Autodesk Fusion 360 part; units mm, degrees
(part 6 of 14)
  arc A1361 (82.693, 15.5542) -> (82.693, 15.6558) centre (82.693, 15.605) ccw
  line L2871 (81.2795, 39.751) -> (80.8045, 39.751)
  arc A1362 (84.693, 13.5542) -> (84.693, 13.6558) centre (84.693, 13.605) ccw
  arc A1363 (82.7386, 13.3061) -> (82.7386, 13.0751) centre (82.7386, 13.1906) ccw
  line L2872 (84.193, 13.3675) -> (84.193, 13.8425)
  line L2873 (81.542, 40.5135) -> (81.542, 40.9885)
  line L2874 (82.042, 39.201) -> (82.042, 40.301)
  line L2875 (83.2795, 40.251) -> (82.8045, 40.251)
  line L2876 (83.2795, 39.251) -> (82.8045, 39.251)
  line L2877 (83.042, 38.751) -> (83.042, 40.751)
  arc A1364 (83.042, 38.7002) -> (83.042, 38.8018) centre (83.042, 38.751) ccw
  line L2878 (81.542, 38.5135) -> (81.542, 38.9885)
  arc A1365 (81.042, 40.7002) -> (81.042, 40.8018) centre (81.042, 40.751) ccw
  line L2879 (82.542, 40.5135) -> (82.542, 40.9885)
  line L2880 (82.542, 38.5135) -> (82.542, 38.9885)
  line L2881 (83.2795, 40.251) -> (82.8045, 40.251)
  arc A1366 (84.693, 13.6558) -> (84.693, 13.5542) centre (84.693, 13.605) ccw
  line L2882 (75.3115, 40.124) -> (75.7865, 40.124)
  line L2883 (82.042, 40.5135) -> (82.042, 40.9885)
  line L2884 (83.2795, 39.251) -> (82.8045, 39.251)
  line L2885 (82.042, 38.5135) -> (82.042, 38.9885)
  line L2886 (83.2795, 39.751) -> (82.8045, 39.751)
  line L2887 (83.2795, 40.251) -> (82.8045, 40.251)
  line L2888 (82.042, 40.5135) -> (82.042, 40.9885)
  line L2889 (82.042, 38.5135) -> (82.042, 38.9885)
  line L2890 (81.542, 40.5135) -> (81.542, 40.9885)
  line L2891 (82.042, 39.201) -> (82.042, 40.301)
  arc A1367 (81.042, 38.7002) -> (81.042, 38.8018) centre (81.042, 38.751) ccw
  line L2892 (83.193, 13.3675) -> (83.193, 13.8425)
  line L2893 (82.542, 38.5135) -> (82.542, 38.9885)
  arc A1368 (83.042, 38.8018) -> (83.042, 38.7002) centre (83.042, 38.751) ccw
  line L2894 (81.2795, 40.251) -> (80.8045, 40.251)
  line L2895 (84.693, 15.605) -> (82.693, 15.605)
  line L2896 (81.2795, 39.751) -> (80.8045, 39.751)
  line L2897 (82.042, 39.201) -> (82.042, 40.301)
  arc A1369 (81.0876, 38.4521) -> (81.0876, 38.2211) centre (81.0876, 38.3366) ccw
  line L2898 (81.542, 40.5135) -> (81.542, 40.9885)
  line L2899 (74.549, 38.8615) -> (74.549, 38.3865)
  line L2900 (81.042, 38.751) -> (83.042, 38.751)
  line L2901 (82.542, 38.5135) -> (82.542, 38.9885)
  line L2902 (81.2795, 39.251) -> (80.8045, 39.251)
  line L2903 (83.693, 13.3675) -> (83.693, 13.8425)
  line L2904 (83.2795, 39.751) -> (82.8045, 39.751)
  line L2905 (73.4385, 13.724) -> (73.9135, 13.724)
  line L2906 (84.9305, 15.105) -> (84.4555, 15.105)
  line L2907 (73.676, 15.224) -> (73.676, 13.224)
  line L2908 (74.676, 15.4615) -> (74.676, 14.9865)
  line L2909 (84.9305, 14.605) -> (84.4555, 14.605)
  arc A1370 (75.676, 15.1732) -> (75.676, 15.2748) centre (75.676, 15.224) ccw
  arc A1371 (73.676, 13.1732) -> (73.676, 13.2748) centre (73.676, 13.224) ccw
  line L2910 (81.2795, 39.751) -> (80.8045, 39.751)
  line L2911 (74.176, 13.4615) -> (74.176, 12.9865)
  line L2912 (82.9305, 14.105) -> (82.4555, 14.105)
  line L2913 (75.676, 13.224) -> (75.676, 15.224)
  line L2914 (83.693, 15.3675) -> (83.693, 15.8425)
  line L2915 (83.693, 13.3675) -> (83.693, 13.8425)
  line L2916 (84.9305, 14.105) -> (84.4555, 14.105)
  line L2917 (83.193, 15.3675) -> (83.193, 15.8425)
  line L2918 (73.4385, 14.724) -> (73.9135, 14.724)
  line L2919 (84.193, 13.3675) -> (84.193, 13.8425)
  line L2920 (84.9305, 14.605) -> (84.4555, 14.605)
  line L2921 (74.176, 15.4615) -> (74.176, 14.9865)
  line L2922 (81.2795, 40.251) -> (80.8045, 40.251)
  arc A1372 (73.676, 13.2748) -> (73.676, 13.1732) centre (73.676, 13.224) ccw
  line L2923 (73.4385, 14.724) -> (73.9135, 14.724)
  arc A1373 (75.676, 15.2748) -> (75.676, 15.1732) centre (75.676, 15.224) ccw
  line L2924 (82.9305, 14.605) -> (82.4555, 14.605)
  line L2925 (74.176, 15.4615) -> (74.176, 14.9865)
  line L2926 (74.176, 15.4615) -> (74.176, 14.9865)
  line L2927 (75.176, 15.4615) -> (75.176, 14.9865)
  arc A1374 (75.676, 13.2748) -> (75.676, 13.1732) centre (75.676, 13.224) ccw
  arc A1375 (73.676, 15.2748) -> (73.676, 15.1732) centre (73.676, 15.224) ccw
  line L2928 (75.176, 15.4615) -> (75.176, 14.9865)
  line L2929 (83.693, 14.055) -> (83.693, 15.155)
  line L2930 (82.693, 13.605) -> (84.693, 13.605)
  line L2931 (82.693, 15.605) -> (82.693, 13.605)
  arc A1376 (73.676, 15.1732) -> (73.676, 15.2748) centre (73.676, 15.224) ccw
  line L2932 (74.676, 15.4615) -> (74.676, 14.9865)
  line L2933 (83.193, 15.3675) -> (83.193, 15.8425)
  line L2934 (83.693, 15.3675) -> (83.693, 15.8425)
  arc A1377 (84.693, 15.6558) -> (84.693, 15.5542) centre (84.693, 15.605) ccw
  line L2935 (84.693, 13.605) -> (84.693, 15.605)
  line L2936 (84.9305, 14.105) -> (84.4555, 14.105)
  line L2937 (84.9305, 14.105) -> (84.4555, 14.105)
  line L2938 (82.9305, 14.105) -> (82.4555, 14.105)
  line L2939 (84.193, 15.3675) -> (84.193, 15.8425)
  line L2940 (83.693, 14.055) -> (83.693, 15.155)
  line L2941 (82.9305, 15.105) -> (82.4555, 15.105)
  line L2942 (84.193, 15.3675) -> (84.193, 15.8425)
  line L2943 (84.9305, 15.105) -> (84.4555, 15.105)
  line L2944 (83.693, 15.3675) -> (83.693, 15.8425)
  line L2945 (84.193, 13.3675) -> (84.193, 13.8425)
  arc A1378 (82.693, 13.5542) -> (82.693, 13.6558) centre (82.693, 13.605) ccw
  line L2946 (84.193, 15.3675) -> (84.193, 15.8425)
  line L2947 (82.9305, 14.105) -> (82.4555, 14.105)
  line L2948 (81.2795, 39.251) -> (80.8045, 39.251)
  line L2949 (84.9305, 14.605) -> (84.4555, 14.605)
  arc A1379 (84.693, 15.5542) -> (84.693, 15.6558) centre (84.693, 15.605) ccw
  line L2950 (82.9305, 15.105) -> (82.4555, 15.105)
  line L2951 (82.9305, 14.605) -> (82.4555, 14.605)
  line L2952 (82.9305, 14.605) -> (82.4555, 14.605)
  line L2953 (84.9305, 15.105) -> (84.4555, 15.105)
  line L2954 (83.693, 14.055) -> (83.693, 15.155)
  line L2955 (83.193, 15.3675) -> (83.193, 15.8425)
  line L2956 (73.4385, 14.224) -> (73.9135, 14.224)
  arc A1380 (82.693, 15.6558) -> (82.693, 15.5542) centre (82.693, 15.605) ccw
  line L2957 (82.9305, 15.105) -> (82.4555, 15.105)
  line L2958 (75.4385, 13.724) -> (75.9135, 13.724)
  line L2959 (92.629, 51.9281) -> (92.629, 52.9281)
  line L2960 (75.4385, 13.724) -> (75.9135, 13.724)
  line L2961 (91.723, 40.621) -> (91.723, 41.001)
  line L2962 (92.173, 39.771) -> (92.173, 40.151)
  line L2963 (92.104, 51.8131) -> (92.104, 52.1931)
  line L2964 (74.676, 15.4615) -> (74.676, 14.9865)
  line L2965 (75.176, 13.4615) -> (75.176, 12.9865)
  arc A1381 (75.6304, 15.7539) -> (75.6304, 15.5229) centre (75.6304, 15.6384) ccw
  line L2966 (92.554, 52.6631) -> (92.554, 53.0431)
  line L2967 (92.029, 52.7281) -> (92.629, 52.7281)
  line L2968 (74.676, 14.774) -> (74.676, 13.674)
  line L2969 (75.4385, 14.224) -> (75.9135, 14.224)
  line L2970 (92.248, 40.886) -> (91.648, 40.886)
  line L2971 (75.676, 15.224) -> (73.676, 15.224)
  line L2972 (74.176, 13.4615) -> (74.176, 12.9865)
  line L2973 (73.4385, 13.724) -> (73.9135, 13.724)
  line L2974 (92.104, 51.8131) -> (92.104, 52.1931)
  line L2975 (91.902, 22.979) -> (91.902, 21.979)
  line L2976 (92.173, 40.621) -> (92.173, 41.001)
  line L2977 (74.676, 13.4615) -> (74.676, 12.9865)
  arc A1382 (92.448, 39.986) -> (92.648, 39.986) centre (92.548, 39.986) ccw
  line L2978 (92.104, 52.6631) -> (92.104, 53.0431)
  line L2979 (91.902, 22.779) -> (92.502, 22.779)
  line L2980 (91.902, 21.979) -> (92.502, 21.979)
  line L2981 (92.104, 51.8131) -> (92.104, 52.1931)
  line L2982 (91.648, 40.686) -> (92.248, 40.686)
  line L2983 (91.723, 40.621) -> (91.723, 41.001)
  line L2984 (73.4385, 14.224) -> (73.9135, 14.224)
  line L2985 (73.4385, 13.724) -> (73.9135, 13.724)
  line L2986 (91.648, 39.886) -> (92.248, 39.886)
  line L2987 (74.676, 13.4615) -> (74.676, 12.9865)
  line L2988 (75.4385, 13.724) -> (75.9135, 13.724)
  line L2989 (75.4385, 14.224) -> (75.9135, 14.224)
  line L2990 (75.4385, 14.724) -> (75.9135, 14.724)
  line L2991 (74.176, 13.4615) -> (74.176, 12.9865)
  line L2992 (74.676, 14.774) -> (74.676, 13.674)
  arc A1383 (75.6304, 15.5229) -> (75.6304, 15.7539) centre (75.6304, 15.6384) ccw
  line L2993 (73.4385, 14.224) -> (73.9135, 14.224)
  line L2994 (73.4385, 14.724) -> (73.9135, 14.724)
  line L2995 (91.648, 40.886) -> (91.648, 39.886)
  arc A1384 (92.648, 39.986) -> (92.448, 39.986) centre (92.548, 39.986) ccw
  line L2996 (92.173, 39.771) -> (92.173, 40.151)
  line L2997 (74.676, 14.774) -> (74.676, 13.674)
  line L2998 (75.176, 13.4615) -> (75.176, 12.9865)
  line L2999 (92.029, 51.9281) -> (92.629, 51.9281)
  line L3000 (92.554, 52.6631) -> (92.554, 53.0431)
  line L3001 (91.723, 39.771) -> (91.723, 40.151)
  arc A1385 (93.029, 52.0281) -> (92.829, 52.0281) centre (92.929, 52.0281) ccw
  line L3002 (92.248, 39.886) -> (92.248, 40.886)
  line L3003 (75.4385, 14.724) -> (75.9135, 14.724)
  arc A1386 (75.676, 13.1732) -> (75.676, 13.2748) centre (75.676, 13.224) ccw
  line L3004 (92.173, 40.621) -> (92.173, 41.001)
  line L3005 (92.554, 52.6631) -> (92.554, 53.0431)
  line L3006 (92.173, 39.771) -> (92.173, 40.151)
  line L3007 (75.4385, 14.724) -> (75.9135, 14.724)
  line L3008 (92.554, 51.8131) -> (92.554, 52.1931)
  line L3009 (75.4385, 14.224) -> (75.9135, 14.224)
  line L3010 (91.648, 40.786) -> (92.248, 40.786)
  line L3011 (75.176, 13.4615) -> (75.176, 12.9865)
  line L3012 (73.676, 13.224) -> (75.676, 13.224)
  line L3013 (74.676, 13.4615) -> (74.676, 12.9865)
  line L3014 (75.176, 15.4615) -> (75.176, 14.9865)
  line L3015 (92.104, 52.6631) -> (92.104, 53.0431)
  arc A1387 (43.735, 39.8716) -> (43.735, 40.1383) centre (43.735, 40.005) ccw
  line L3016 (62.005, 17.735) -> (38.465, 17.735)
  arc A1388 (40.735, 39.8716) -> (40.735, 40.1383) centre (40.735, 40.005) ccw
  arc A1389 (37.8892, 40.2746) -> (37.2672, 40.2746) centre (37.5782, 40.2746) ccw
  arc A1390 (39.2088, 40.0206) -> (40.2656, 40.0206) centre (39.7372, 40.0206) ccw
  arc A1391 (92.829, 52.0281) -> (93.029, 52.0281) centre (92.929, 52.0281) ccw
  arc A1392 (42.735, 39.8716) -> (42.735, 40.1383) centre (42.735, 40.005) ccw
  arc A1393 (39.735, 40.1383) -> (39.735, 39.8717) centre (39.735, 40.005) ccw
  line L3017 (64.205, 15.535) -> (64.205, 43.475)
  arc A1394 (41.735, 40.1383) -> (41.735, 39.8717) centre (41.735, 40.005) ccw
  line L3018 (91.723, 39.771) -> (91.723, 40.151)
  line L3019 (92.104, 52.6631) -> (92.104, 53.0431)
  line L3020 (92.502, 22.979) -> (91.902, 22.979)
  line L3021 (92.681, 7.767) -> (92.681, 8.147)
  line L3022 (92.156, 8.682) -> (92.756, 8.682)
  line L3023 (91.723, 39.771) -> (91.723, 40.151)
  line L3024 (92.156, 8.882) -> (92.156, 7.882)
  line L3025 (92.756, 8.882) -> (92.156, 8.882)
  line L3026 (92.427, 21.864) -> (92.427, 22.244)
  line L3027 (92.681, 8.617) -> (92.681, 8.997)
  line L3028 (92.681, 7.767) -> (92.681, 8.147)
  line L3029 (92.427, 22.714) -> (92.427, 23.094)
  line L3030 (92.156, 8.782) -> (92.756, 8.782)
  line L3031 (92.756, 7.882) -> (92.756, 8.882)
  line L3032 (92.681, 8.617) -> (92.681, 8.997)
  arc A1395 (40.735, 39.8716) -> (40.735, 40.1383) centre (40.735, 40.005) ccw
  line L3033 (92.173, 40.621) -> (92.173, 41.001)
  line L3034 (92.681, 8.617) -> (92.681, 8.997)
  line L3035 (92.502, 21.979) -> (92.502, 22.979)
  arc A1396 (42.735, 39.8716) -> (42.735, 40.1383) centre (42.735, 40.005) ccw
  arc A1397 (92.956, 7.982) -> (93.156, 7.982) centre (93.056, 7.982) ccw
  line L3036 (92.029, 52.9281) -> (92.029, 51.9281)
  line L3037 (91.977, 21.864) -> (91.977, 22.244)
  line L3038 (92.231, 8.617) -> (92.231, 8.997)
  arc A1398 (41.735, 40.1383) -> (41.735, 39.8717) centre (41.735, 40.005) ccw
  line L3039 (92.156, 7.882) -> (92.756, 7.882)
  line L3040 (91.977, 21.864) -> (91.977, 22.244)
  line L3041 (64.205, 43.475) -> (36.265, 43.475)
  line L3042 (91.977, 22.714) -> (91.977, 23.094)
  line L3043 (92.231, 7.767) -> (92.231, 8.147)
  line L3044 (36.265, 15.535) -> (64.205, 15.535)
  arc A1399 (92.702, 22.079) -> (92.902, 22.079) centre (92.802, 22.079) ccw
  arc A1400 (41.735, 39.8716) -> (41.735, 40.1383) centre (41.735, 40.005) ccw
  line L3045 (91.723, 40.621) -> (91.723, 41.001)
  line L3046 (92.427, 21.864) -> (92.427, 22.244)
  line L3047 (91.902, 22.879) -> (92.502, 22.879)
  line L3048 (92.427, 22.714) -> (92.427, 23.094)
  line L3049 (92.681, 7.767) -> (92.681, 8.147)
  line L3050 (92.231, 8.617) -> (92.231, 8.997)
  arc A1401 (40.735, 40.1383) -> (40.735, 39.8717) centre (40.735, 40.005) ccw
  line L3051 (92.554, 51.8131) -> (92.554, 52.1931)
  line L3052 (92.231, 7.767) -> (92.231, 8.147)
  line L3053 (92.554, 51.8131) -> (92.554, 52.1931)
  arc A1402 (92.902, 22.079) -> (92.702, 22.079) centre (92.802, 22.079) ccw
  line L3054 (91.977, 22.714) -> (91.977, 23.094)
  line L3055 (92.427, 21.864) -> (92.427, 22.244)
  line L3056 (92.029, 52.8281) -> (92.629, 52.8281)
  line L3057 (91.977, 22.714) -> (91.977, 23.094)
  line L3058 (92.231, 8.617) -> (92.231, 8.997)
  arc A1403 (93.156, 7.982) -> (92.956, 7.982) centre (93.056, 7.982) ccw
  line L3059 (92.427, 22.714) -> (92.427, 23.094)
  line L3060 (48.395, 52.0775) -> (48.395, 54.3505)
  line L3061 (91.977, 21.864) -> (91.977, 22.244)
  line L3062 (92.629, 52.9281) -> (92.029, 52.9281)
  arc A1404 (44.735, 40.1383) -> (44.735, 39.8717) centre (44.735, 40.005) ccw
  arc A1405 (46.735, 39.8716) -> (46.735, 40.1383) centre (46.735, 40.005) ccw
  arc A1406 (48.735, 39.8716) -> (48.735, 40.1383) centre (48.735, 40.005) ccw
  arc A1407 (43.735, 39.8716) -> (43.735, 40.1383) centre (43.735, 40.005) ccw
  arc A1408 (47.735, 40.1383) -> (47.735, 39.8717) centre (47.735, 40.005) ccw
  arc A1409 (48.735, 40.1383) -> (48.735, 39.8717) centre (48.735, 40.005) ccw
  arc A1410 (43.735, 39.8716) -> (43.735, 40.1383) centre (43.735, 40.005) ccw
  arc A1411 (45.735, 39.8716) -> (45.735, 40.1383) centre (45.735, 40.005) ccw
  arc A1412 (45.735, 39.8716) -> (45.735, 40.1383) centre (45.735, 40.005) ccw
  arc A1413 (41.735, 39.8716) -> (41.735, 40.1383) centre (41.735, 40.005) ccw
  arc A1414 (47.735, 40.1383) -> (47.735, 39.8717) centre (47.735, 40.005) ccw
  arc A1415 (47.735, 39.8716) -> (47.735, 40.1383) centre (47.735, 40.005) ccw
  arc A1416 (42.735, 40.1383) -> (42.735, 39.8717) centre (42.735, 40.005) ccw
  arc A1417 (45.735, 40.1383) -> (45.735, 39.8717) centre (45.735, 40.005) ccw
  arc A1418 (43.735, 40.1383) -> (43.735, 39.8717) centre (43.735, 40.005) ccw
  arc A1419 (45.735, 40.1383) -> (45.735, 39.8717) centre (45.735, 40.005) ccw
  arc A1420 (37.2672, 40.2746) -> (37.8892, 40.2746) centre (37.5782, 40.2746) ccw
  arc A1421 (48.735, 39.8716) -> (48.735, 40.1383) centre (48.735, 40.005) ccw
  arc A1422 (49.735, 39.8716) -> (49.735, 40.1383) centre (49.735, 40.005) ccw
  arc A1423 (39.735, 39.8716) -> (39.735, 40.1383) centre (39.735, 40.005) ccw
  line L3063 (38.465, 17.735) -> (38.465, 41.275)
  arc A1424 (44.735, 40.1383) -> (44.735, 39.8717) centre (44.735, 40.005) ccw
  arc A1425 (39.735, 40.1383) -> (39.735, 39.8717) centre (39.735, 40.005) ccw
  arc A1426 (44.735, 39.8716) -> (44.735, 40.1383) centre (44.735, 40.005) ccw
  arc A1427 (49.735, 40.1383) -> (49.735, 39.8717) centre (49.735, 40.005) ccw
  arc A1428 (45.735, 40.1383) -> (45.735, 39.8717) centre (45.735, 40.005) ccw
  arc A1429 (46.735, 40.1383) -> (46.735, 39.8717) centre (46.735, 40.005) ccw
  arc A1430 (49.735, 39.8716) -> (49.735, 40.1383) centre (49.735, 40.005) ccw
  arc A1431 (42.735, 40.1383) -> (42.735, 39.8717) centre (42.735, 40.005) ccw
  arc A1432 (49.735, 40.1383) -> (49.735, 39.8717) centre (49.735, 40.005) ccw
  arc A1433 (49.735, 39.8716) -> (49.735, 40.1383) centre (49.735, 40.005) ccw
  arc A1434 (48.735, 40.1383) -> (48.735, 39.8717) centre (48.735, 40.005) ccw
  arc A1435 (46.735, 39.8716) -> (46.735, 40.1383) centre (46.735, 40.005) ccw
  arc A1436 (46.735, 40.1383) -> (46.735, 39.8717) centre (46.735, 40.005) ccw
  arc A1437 (40.735, 40.1383) -> (40.735, 39.8717) centre (40.735, 40.005) ccw
  arc A1438 (50.735, 39.8716) -> (50.735, 40.1383) centre (50.735, 40.005) ccw
  arc A1439 (44.735, 39.8716) -> (44.735, 40.1383) centre (44.735, 40.005) ccw
  arc A1440 (47.735, 39.8716) -> (47.735, 40.1383) centre (47.735, 40.005) ccw
  arc A1441 (48.735, 39.8716) -> (48.735, 40.1383) centre (48.735, 40.005) ccw
  arc A1442 (40.735, 39.8716) -> (40.735, 40.1383) centre (40.735, 40.005) ccw
  line L3064 (92.231, 7.767) -> (92.231, 8.147)
  arc A1443 (41.735, 40.1383) -> (41.735, 39.8717) centre (41.735, 40.005) ccw
  line L3065 (62.005, 41.275) -> (62.005, 17.735)
  arc A1444 (42.735, 39.8716) -> (42.735, 40.1383) centre (42.735, 40.005) ccw
  arc A1445 (43.735, 40.1383) -> (43.735, 39.8717) centre (43.735, 40.005) ccw
  arc A1446 (45.735, 39.8716) -> (45.735, 40.1383) centre (45.735, 40.005) ccw
  line L3066 (36.265, 43.475) -> (36.265, 15.535)
  arc A1447 (46.735, 40.1383) -> (46.735, 39.8717) centre (46.735, 40.005) ccw
  arc A1448 (40.2656, 40.0206) -> (39.2088, 40.0206) centre (39.7372, 40.0206) ccw
  arc A1449 (47.735, 39.8716) -> (47.735, 40.1383) centre (47.735, 40.005) ccw
  arc A1450 (41.735, 39.8716) -> (41.735, 40.1383) centre (41.735, 40.005) ccw
  arc A1451 (39.735, 39.8716) -> (39.735, 40.1383) centre (39.735, 40.005) ccw
  arc A1452 (42.735, 40.1383) -> (42.735, 39.8717) centre (42.735, 40.005) ccw
  arc A1453 (43.735, 40.1383) -> (43.735, 39.8717) centre (43.735, 40.005) ccw
  arc A1454 (40.735, 40.1383) -> (40.735, 39.8717) centre (40.735, 40.005) ccw
  arc A1455 (49.735, 40.1383) -> (49.735, 39.8717) centre (49.735, 40.005) ccw
  arc A1456 (48.735, 40.1383) -> (48.735, 39.8717) centre (48.735, 40.005) ccw
  arc A1457 (44.735, 39.8716) -> (44.735, 40.1383) centre (44.735, 40.005) ccw
  arc A1458 (44.735, 40.1383) -> (44.735, 39.8717) centre (44.735, 40.005) ccw
  arc A1459 (39.735, 39.8716) -> (39.735, 40.1383) centre (39.735, 40.005) ccw
  arc A1460 (39.735, 40.1383) -> (39.735, 39.8717) centre (39.735, 40.005) ccw
  line L3067 (38.465, 41.275) -> (62.005, 41.275)
  arc A1461 (46.735, 39.8716) -> (46.735, 40.1383) centre (46.735, 40.005) ccw
  arc A1462 (47.735, 40.1383) -> (47.735, 39.8717) centre (47.735, 40.005) ccw
  arc A1463 (59.735, 39.8716) -> (59.735, 40.1383) centre (59.735, 40.005) ccw
  arc A1464 (56.735, 40.1383) -> (56.735, 39.8717) centre (56.735, 40.005) ccw
  arc A1465 (58.735, 40.1383) -> (58.735, 39.8717) centre (58.735, 40.005) ccw
  arc A1466 (59.735, 40.1383) -> (59.735, 39.8717) centre (59.735, 40.005) ccw
  arc A1467 (51.735, 40.1383) -> (51.735, 39.8717) centre (51.735, 40.005) ccw
  arc A1468 (53.735, 40.1383) -> (53.735, 39.8717) centre (53.735, 40.005) ccw
  arc A1469 (53.735, 39.8716) -> (53.735, 40.1383) centre (53.735, 40.005) ccw
  arc A1470 (55.735, 39.8716) -> (55.735, 40.1383) centre (55.735, 40.005) ccw
  arc A1471 (60.735, 39.8716) -> (60.735, 40.1383) centre (60.735, 40.005) ccw
  arc A1472 (59.735, 39.8716) -> (59.735, 40.1383) centre (59.735, 40.005) ccw
  arc A1473 (51.735, 40.1383) -> (51.735, 39.8717) centre (51.735, 40.005) ccw
  arc A1474 (58.735, 39.8716) -> (58.735, 40.1383) centre (58.735, 40.005) ccw
  arc A1475 (54.735, 39.8716) -> (54.735, 40.1383) centre (54.735, 40.005) ccw
  arc A1476 (56.735, 40.1383) -> (56.735, 39.8717) centre (56.735, 40.005) ccw
  arc A1477 (59.735, 39.8716) -> (59.735, 40.1383) centre (59.735, 40.005) ccw
  arc A1478 (52.735, 39.8716) -> (52.735, 40.1383) centre (52.735, 40.005) ccw
  arc A1479 (54.735, 40.1383) -> (54.735, 39.8717) centre (54.735, 40.005) ccw
  arc A1480 (58.735, 39.8716) -> (58.735, 40.1383) centre (58.735, 40.005) ccw
  arc A1481 (54.735, 40.1383) -> (54.735, 39.8717) centre (54.735, 40.005) ccw
  arc A1482 (60.735, 40.1383) -> (60.735, 39.8717) centre (60.735, 40.005) ccw
  arc A1483 (58.735, 40.1383) -> (58.735, 39.8717) centre (58.735, 40.005) ccw
  arc A1484 (50.735, 39.8716) -> (50.735, 40.1383) centre (50.735, 40.005) ccw
  arc A1485 (55.735, 40.1383) -> (55.735, 39.8717) centre (55.735, 40.005) ccw
  arc A1486 (57.735, 39.8716) -> (57.735, 40.1383) centre (57.735, 40.005) ccw
  arc A1487 (60.735, 40.1383) -> (60.735, 39.8717) centre (60.735, 40.005) ccw
  arc A1488 (56.735, 39.8716) -> (56.735, 40.1383) centre (56.735, 40.005) ccw
  arc A1489 (59.735, 40.1383) -> (59.735, 39.8717) centre (59.735, 40.005) ccw
  arc A1490 (56.735, 39.8716) -> (56.735, 40.1383) centre (56.735, 40.005) ccw
  arc A1491 (55.735, 39.8716) -> (55.735, 40.1383) centre (55.735, 40.005) ccw
  arc A1492 (56.735, 40.1383) -> (56.735, 39.8717) centre (56.735, 40.005) ccw
  arc A1493 (58.735, 40.1383) -> (58.735, 39.8717) centre (58.735, 40.005) ccw
  arc A1494 (59.735, 40.1383) -> (59.735, 39.8717) centre (59.735, 40.005) ccw
  arc A1495 (60.735, 39.8716) -> (60.735, 40.1383) centre (60.735, 40.005) ccw
  arc A1496 (39.735, 38.8716) -> (39.735, 39.1383) centre (39.735, 39.005) ccw
  arc A1497 (58.735, 39.8716) -> (58.735, 40.1383) centre (58.735, 40.005) ccw
  arc A1498 (55.735, 39.8716) -> (55.735, 40.1383) centre (55.735, 40.005) ccw
  arc A1499 (50.735, 39.8716) -> (50.735, 40.1383) centre (50.735, 40.005) ccw
  arc A1500 (53.735, 40.1383) -> (53.735, 39.8717) centre (53.735, 40.005) ccw
  arc A1501 (52.735, 39.8716) -> (52.735, 40.1383) centre (52.735, 40.005) ccw
  arc A1502 (54.735, 39.8716) -> (54.735, 40.1383) centre (54.735, 40.005) ccw
  arc A1503 (52.735, 40.1383) -> (52.735, 39.8717) centre (52.735, 40.005) ccw
  arc A1504 (51.735, 40.1383) -> (51.735, 39.8717) centre (51.735, 40.005) ccw
  arc A1505 (52.735, 40.1383) -> (52.735, 39.8717) centre (52.735, 40.005) ccw
  arc A1506 (53.735, 40.1383) -> (53.735, 39.8717) centre (53.735, 40.005) ccw
  arc A1507 (52.735, 40.1383) -> (52.735, 39.8717) centre (52.735, 40.005) ccw
  arc A1508 (51.735, 39.8716) -> (51.735, 40.1383) centre (51.735, 40.005) ccw
  arc A1509 (55.735, 40.1383) -> (55.735, 39.8717) centre (55.735, 40.005) ccw
  arc A1510 (51.735, 39.8716) -> (51.735, 40.1383) centre (51.735, 40.005) ccw
  arc A1511 (53.735, 39.8716) -> (53.735, 40.1383) centre (53.735, 40.005) ccw
  arc A1512 (50.735, 40.1383) -> (50.735, 39.8717) centre (50.735, 40.005) ccw
  arc A1513 (54.735, 40.1383) -> (54.735, 39.8717) centre (54.735, 40.005) ccw
  arc A1514 (50.735, 40.1383) -> (50.735, 39.8717) centre (50.735, 40.005) ccw
  arc A1515 (53.735, 39.8716) -> (53.735, 40.1383) centre (53.735, 40.005) ccw
  arc A1516 (51.735, 39.8716) -> (51.735, 40.1383) centre (51.735, 40.005) ccw
  arc A1517 (54.735, 39.8716) -> (54.735, 40.1383) centre (54.735, 40.005) ccw
  arc A1518 (52.735, 39.8716) -> (52.735, 40.1383) centre (52.735, 40.005) ccw
  arc A1519 (56.735, 39.8716) -> (56.735, 40.1383) centre (56.735, 40.005) ccw
  arc A1520 (39.735, 39.1383) -> (39.735, 38.8716) centre (39.735, 39.005) ccw
  arc A1521 (57.735, 39.8716) -> (57.735, 40.1383) centre (57.735, 40.005) ccw
  arc A1522 (57.735, 39.8716) -> (57.735, 40.1383) centre (57.735, 40.005) ccw
  arc A1523 (55.735, 40.1383) -> (55.735, 39.8717) centre (55.735, 40.005) ccw
  arc A1524 (57.735, 40.1383) -> (57.735, 39.8717) centre (57.735, 40.005) ccw
  arc A1525 (50.735, 40.1383) -> (50.735, 39.8717) centre (50.735, 40.005) ccw
  arc A1526 (57.735, 40.1383) -> (57.735, 39.8717) centre (57.735, 40.005) ccw
  arc A1527 (41.735, 39.1383) -> (41.735, 38.8716) centre (41.735, 39.005) ccw
  arc A1528 (40.735, 39.1383) -> (40.735, 38.8716) centre (40.735, 39.005) ccw
  arc A1529 (60.735, 40.1383) -> (60.735, 39.8717) centre (60.735, 40.005) ccw
  arc A1530 (45.735, 38.8716) -> (45.735, 39.1383) centre (45.735, 39.005) ccw
  arc A1531 (45.735, 38.8716) -> (45.735, 39.1383) centre (45.735, 39.005) ccw
  arc A1532 (42.735, 39.1383) -> (42.735, 38.8716) centre (42.735, 39.005) ccw
  arc A1533 (41.735, 39.1383) -> (41.735, 38.8716) centre (41.735, 39.005) ccw
  arc A1534 (42.735, 38.8716) -> (42.735, 39.1383) centre (42.735, 39.005) ccw
  arc A1535 (42.735, 39.1383) -> (42.735, 38.8716) centre (42.735, 39.005) ccw
  arc A1536 (46.735, 38.8716) -> (46.735, 39.1383) centre (46.735, 39.005) ccw
  arc A1537 (40.735, 38.8716) -> (40.735, 39.1383) centre (40.735, 39.005) ccw
  arc A1538 (40.735, 38.8716) -> (40.735, 39.1383) centre (40.735, 39.005) ccw
  arc A1539 (43.735, 38.8716) -> (43.735, 39.1383) centre (43.735, 39.005) ccw
  arc A1540 (43.735, 39.1383) -> (43.735, 38.8716) centre (43.735, 39.005) ccw
  arc A1541 (48.735, 39.1383) -> (48.735, 38.8716) centre (48.735, 39.005) ccw
  arc A1542 (45.735, 39.1383) -> (45.735, 38.8716) centre (45.735, 39.005) ccw
  arc A1543 (41.735, 38.8716) -> (41.735, 39.1383) centre (41.735, 39.005) ccw
  arc A1544 (49.735, 39.1383) -> (49.735, 38.8716) centre (49.735, 39.005) ccw
  arc A1545 (48.735, 38.8716) -> (48.735, 39.1383) centre (48.735, 39.005) ccw
  arc A1546 (47.735, 39.1383) -> (47.735, 38.8716) centre (47.735, 39.005) ccw
  arc A1547 (49.735, 39.1383) -> (49.735, 38.8716) centre (49.735, 39.005) ccw
  arc A1548 (46.735, 39.1383) -> (46.735, 38.8716) centre (46.735, 39.005) ccw
  arc A1549 (49.735, 38.8716) -> (49.735, 39.1383) centre (49.735, 39.005) ccw
  arc A1550 (45.735, 38.8716) -> (45.735, 39.1383) centre (45.735, 39.005) ccw
  arc A1551 (47.735, 38.8716) -> (47.735, 39.1383) centre (47.735, 39.005) ccw
  arc A1552 (50.735, 39.1383) -> (50.735, 38.8716) centre (50.735, 39.005) ccw
  arc A1553 (60.735, 39.8716) -> (60.735, 40.1383) centre (60.735, 40.005) ccw
  arc A1554 (50.735, 38.8716) -> (50.735, 39.1383) centre (50.735, 39.005) ccw
  arc A1555 (51.735, 38.8716) -> (51.735, 39.1383) centre (51.735, 39.005) ccw
  arc A1556 (40.735, 38.8716) -> (40.735, 39.1383) centre (40.735, 39.005) ccw
  arc A1557 (48.735, 39.1383) -> (48.735, 38.8716) centre (48.735, 39.005) ccw
  arc A1558 (49.735, 38.8716) -> (49.735, 39.1383) centre (49.735, 39.005) ccw
  arc A1559 (50.735, 38.8716) -> (50.735, 39.1383) centre (50.735, 39.005) ccw
  arc A1560 (47.735, 39.1383) -> (47.735, 38.8716) centre (47.735, 39.005) ccw
  arc A1561 (51.735, 39.1383) -> (51.735, 38.8716) centre (51.735, 39.005) ccw
  arc A1562 (43.735, 38.8716) -> (43.735, 39.1383) centre (43.735, 39.005) ccw
  arc A1563 (57.735, 40.1383) -> (57.735, 39.8717) centre (57.735, 40.005) ccw
  arc A1564 (39.735, 39.1383) -> (39.735, 38.8716) centre (39.735, 39.005) ccw
  arc A1565 (46.735, 39.1383) -> (46.735, 38.8716) centre (46.735, 39.005) ccw
  arc A1566 (42.735, 38.8716) -> (42.735, 39.1383) centre (42.735, 39.005) ccw
  arc A1567 (45.735, 39.1383) -> (45.735, 38.8716) centre (45.735, 39.005) ccw
  arc A1568 (41.735, 38.8716) -> (41.735, 39.1383) centre (41.735, 39.005) ccw
  arc A1569 (46.735, 39.1383) -> (46.735, 38.8716) centre (46.735, 39.005) ccw
  arc A1570 (43.735, 39.1383) -> (43.735, 38.8716) centre (43.735, 39.005) ccw
  arc A1571 (43.735, 39.1383) -> (43.735, 38.8716) centre (43.735, 39.005) ccw
  arc A1572 (40.735, 39.1383) -> (40.735, 38.8716) centre (40.735, 39.005) ccw
  arc A1573 (46.735, 38.8716) -> (46.735, 39.1383) centre (46.735, 39.005) ccw
  arc A1574 (44.735, 39.1383) -> (44.735, 38.8716) centre (44.735, 39.005) ccw
  arc A1575 (41.735, 38.8716) -> (41.735, 39.1383) centre (41.735, 39.005) ccw
  arc A1576 (39.735, 38.8716) -> (39.735, 39.1383) centre (39.735, 39.005) ccw
  arc A1577 (44.735, 38.8716) -> (44.735, 39.1383) centre (44.735, 39.005) ccw
  arc A1578 (42.735, 38.8716) -> (42.735, 39.1383) centre (42.735, 39.005) ccw
  arc A1579 (43.735, 38.8716) -> (43.735, 39.1383) centre (43.735, 39.005) ccw
  arc A1580 (44.735, 38.8716) -> (44.735, 39.1383) centre (44.735, 39.005) ccw
  arc A1581 (39.735, 39.1383) -> (39.735, 38.8716) centre (39.735, 39.005) ccw
  arc A1582 (39.735, 38.8716) -> (39.735, 39.1383) centre (39.735, 39.005) ccw
  arc A1583 (45.735, 39.1383) -> (45.735, 38.8716) centre (45.735, 39.005) ccw
  arc A1584 (44.735, 38.8716) -> (44.735, 39.1383) centre (44.735, 39.005) ccw
  arc A1585 (40.735, 39.1383) -> (40.735, 38.8716) centre (40.735, 39.005) ccw
  arc A1586 (44.735, 39.1383) -> (44.735, 38.8716) centre (44.735, 39.005) ccw
  arc A1587 (46.735, 38.8716) -> (46.735, 39.1383) centre (46.735, 39.005) ccw
  arc A1588 (41.735, 39.1383) -> (41.735, 38.8716) centre (41.735, 39.005) ccw
  arc A1589 (44.735, 39.1383) -> (44.735, 38.8716) centre (44.735, 39.005) ccw
  arc A1590 (42.735, 39.1383) -> (42.735, 38.8716) centre (42.735, 39.005) ccw
  arc A1591 (50.735, 39.1383) -> (50.735, 38.8716) centre (50.735, 39.005) ccw
  arc A1592 (55.735, 39.1383) -> (55.735, 38.8716) centre (55.735, 39.005) ccw
  arc A1593 (58.735, 38.8716) -> (58.735, 39.1383) centre (58.735, 39.005) ccw
  arc A1594 (58.735, 39.1383) -> (58.735, 38.8716) centre (58.735, 39.005) ccw
  arc A1595 (58.735, 38.8716) -> (58.735, 39.1383) centre (58.735, 39.005) ccw
  arc A1596 (53.735, 39.1383) -> (53.735, 38.8716) centre (53.735, 39.005) ccw
  arc A1597 (59.735, 38.8716) -> (59.735, 39.1383) centre (59.735, 39.005) ccw
  arc A1598 (59.735, 39.1383) -> (59.735, 38.8716) centre (59.735, 39.005) ccw
  arc A1599 (52.735, 39.1383) -> (52.735, 38.8716) centre (52.735, 39.005) ccw
  arc A1600 (59.735, 39.1383) -> (59.735, 38.8716) centre (59.735, 39.005) ccw
  arc A1601 (59.735, 39.1383) -> (59.735, 38.8716) centre (59.735, 39.005) ccw
  arc A1602 (50.735, 39.1383) -> (50.735, 38.8716) centre (50.735, 39.005) ccw
  arc A1603 (55.735, 39.1383) -> (55.735, 38.8716) centre (55.735, 39.005) ccw
  arc A1604 (51.735, 38.8716) -> (51.735, 39.1383) centre (51.735, 39.005) ccw
  arc A1605 (52.735, 38.8716) -> (52.735, 39.1383) centre (52.735, 39.005) ccw
  arc A1606 (54.735, 39.1383) -> (54.735, 38.8716) centre (54.735, 39.005) ccw
  arc A1607 (54.735, 39.1383) -> (54.735, 38.8716) centre (54.735, 39.005) ccw
  arc A1608 (54.735, 38.8716) -> (54.735, 39.1383) centre (54.735, 39.005) ccw
  arc A1609 (57.735, 39.1383) -> (57.735, 38.8716) centre (57.735, 39.005) ccw
  arc A1610 (59.735, 38.8716) -> (59.735, 39.1383) centre (59.735, 39.005) ccw
  arc A1611 (53.735, 38.8716) -> (53.735, 39.1383) centre (53.735, 39.005) ccw
  arc A1612 (47.735, 38.8716) -> (47.735, 39.1383) centre (47.735, 39.005) ccw
  arc A1613 (48.735, 38.8716) -> (48.735, 39.1383) centre (48.735, 39.005) ccw
  arc A1614 (58.735, 38.8716) -> (58.735, 39.1383) centre (58.735, 39.005) ccw
  arc A1615 (59.735, 38.8716) -> (59.735, 39.1383) centre (59.735, 39.005) ccw
  arc A1616 (55.735, 38.8716) -> (55.735, 39.1383) centre (55.735, 39.005) ccw
  arc A1617 (57.735, 39.1383) -> (57.735, 38.8716) centre (57.735, 39.005) ccw
  arc A1618 (58.735, 39.1383) -> (58.735, 38.8716) centre (58.735, 39.005) ccw
  arc A1619 (60.735, 39.1383) -> (60.735, 38.8716) centre (60.735, 39.005) ccw
  arc A1620 (56.735, 38.8716) -> (56.735, 39.1383) centre (56.735, 39.005) ccw
  arc A1621 (51.735, 39.1383) -> (51.735, 38.8716) centre (51.735, 39.005) ccw
  arc A1622 (49.735, 38.8716) -> (49.735, 39.1383) centre (49.735, 39.005) ccw
  arc A1623 (57.735, 38.8716) -> (57.735, 39.1383) centre (57.735, 39.005) ccw
  arc A1624 (53.735, 38.8716) -> (53.735, 39.1383) centre (53.735, 39.005) ccw
  arc A1625 (52.735, 38.8716) -> (52.735, 39.1383) centre (52.735, 39.005) ccw
  arc A1626 (54.735, 39.1383) -> (54.735, 38.8716) centre (54.735, 39.005) ccw
  arc A1627 (52.735, 39.1383) -> (52.735, 38.8716) centre (52.735, 39.005) ccw
  arc A1628 (48.735, 39.1383) -> (48.735, 38.8716) centre (48.735, 39.005) ccw
  arc A1629 (54.735, 38.8716) -> (54.735, 39.1383) centre (54.735, 39.005) ccw
  arc A1630 (51.735, 39.1383) -> (51.735, 38.8716) centre (51.735, 39.005) ccw
  arc A1631 (56.735, 39.1383) -> (56.735, 38.8716) centre (56.735, 39.005) ccw
  arc A1632 (57.735, 39.1383) -> (57.735, 38.8716) centre (57.735, 39.005) ccw
  arc A1633 (47.735, 39.1383) -> (47.735, 38.8716) centre (47.735, 39.005) ccw
  arc A1634 (49.735, 39.1383) -> (49.735, 38.8716) centre (49.735, 39.005) ccw
  arc A1635 (55.735, 38.8716) -> (55.735, 39.1383) centre (55.735, 39.005) ccw
  arc A1636 (54.735, 38.8716) -> (54.735, 39.1383) centre (54.735, 39.005) ccw
  arc A1637 (47.735, 38.8716) -> (47.735, 39.1383) centre (47.735, 39.005) ccw
  arc A1638 (57.735, 38.8716) -> (57.735, 39.1383) centre (57.735, 39.005) ccw
  arc A1639 (56.735, 39.1383) -> (56.735, 38.8716) centre (56.735, 39.005) ccw
  arc A1640 (53.735, 38.8716) -> (53.735, 39.1383) centre (53.735, 39.005) ccw
  arc A1641 (55.735, 38.8716) -> (55.735, 39.1383) centre (55.735, 39.005) ccw
  arc A1642 (52.735, 39.1383) -> (52.735, 38.8716) centre (52.735, 39.005) ccw
  arc A1643 (56.735, 38.8716) -> (56.735, 39.1383) centre (56.735, 39.005) ccw
  arc A1644 (58.735, 39.1383) -> (58.735, 38.8716) centre (58.735, 39.005) ccw
  arc A1645 (50.735, 38.8716) -> (50.735, 39.1383) centre (50.735, 39.005) ccw
  arc A1646 (48.735, 38.8716) -> (48.735, 39.1383) centre (48.735, 39.005) ccw
  arc A1647 (55.735, 39.1383) -> (55.735, 38.8716) centre (55.735, 39.005) ccw
  arc A1648 (53.735, 39.1383) -> (53.735, 38.8716) centre (53.735, 39.005) ccw
  arc A1649 (52.735, 38.8716) -> (52.735, 39.1383) centre (52.735, 39.005) ccw
  arc A1650 (53.735, 39.1383) -> (53.735, 38.8716) centre (53.735, 39.005) ccw
  arc A1651 (56.735, 38.8716) -> (56.735, 39.1383) centre (56.735, 39.005) ccw
  arc A1652 (57.735, 38.8716) -> (57.735, 39.1383) centre (57.735, 39.005) ccw
  arc A1653 (51.735, 38.8716) -> (51.735, 39.1383) centre (51.735, 39.005) ccw
  arc A1654 (56.735, 39.1383) -> (56.735, 38.8716) centre (56.735, 39.005) ccw
  arc A1655 (48.735, 38.1383) -> (48.735, 37.8716) centre (48.735, 38.005) ccw
  arc A1656 (41.735, 38.1383) -> (41.735, 37.8716) centre (41.735, 38.005) ccw
  arc A1657 (49.735, 38.1383) -> (49.735, 37.8716) centre (49.735, 38.005) ccw
  arc A1658 (60.735, 38.8716) -> (60.735, 39.1383) centre (60.735, 39.005) ccw
  arc A1659 (47.735, 37.8716) -> (47.735, 38.1383) centre (47.735, 38.005) ccw
  arc A1660 (45.735, 37.8716) -> (45.735, 38.1383) centre (45.735, 38.005) ccw
  arc A1661 (41.735, 37.8716) -> (41.735, 38.1383) centre (41.735, 38.005) ccw
  arc A1662 (40.735, 38.1383) -> (40.735, 37.8716) centre (40.735, 38.005) ccw
  arc A1663 (50.735, 37.8716) -> (50.735, 38.1383) centre (50.735, 38.005) ccw
  arc A1664 (46.735, 38.1383) -> (46.735, 37.8716) centre (46.735, 38.005) ccw
  arc A1665 (48.735, 38.1383) -> (48.735, 37.8716) centre (48.735, 38.005) ccw
  arc A1666 (44.735, 37.8716) -> (44.735, 38.1383) centre (44.735, 38.005) ccw
  arc A1667 (43.735, 38.1383) -> (43.735, 37.8716) centre (43.735, 38.005) ccw
  arc A1668 (40.735, 37.8716) -> (40.735, 38.1383) centre (40.735, 38.005) ccw
  arc A1669 (40.735, 37.8716) -> (40.735, 38.1383) centre (40.735, 38.005) ccw
  arc A1670 (48.735, 37.8716) -> (48.735, 38.1383) centre (48.735, 38.005) ccw
  arc A1671 (39.735, 37.8716) -> (39.735, 38.1383) centre (39.735, 38.005) ccw
  arc A1672 (48.735, 38.1383) -> (48.735, 37.8716) centre (48.735, 38.005) ccw
  arc A1673 (39.735, 38.1383) -> (39.735, 37.8716) centre (39.735, 38.005) ccw
  arc A1674 (41.735, 37.8716) -> (41.735, 38.1383) centre (41.735, 38.005) ccw
  arc A1675 (60.735, 38.8716) -> (60.735, 39.1383) centre (60.735, 39.005) ccw
  arc A1676 (49.735, 37.8716) -> (49.735, 38.1383) centre (49.735, 38.005) ccw
  arc A1677 (49.735, 37.8716) -> (49.735, 38.1383) centre (49.735, 38.005) ccw
  arc A1678 (43.735, 37.8716) -> (43.735, 38.1383) centre (43.735, 38.005) ccw
  arc A1679 (44.735, 37.8716) -> (44.735, 38.1383) centre (44.735, 38.005) ccw
  arc A1680 (45.735, 38.1383) -> (45.735, 37.8716) centre (45.735, 38.005) ccw
  arc A1681 (49.735, 38.1383) -> (49.735, 37.8716) centre (49.735, 38.005) ccw
  arc A1682 (49.735, 38.1383) -> (49.735, 37.8716) centre (49.735, 38.005) ccw
  arc A1683 (46.735, 38.1383) -> (46.735, 37.8716) centre (46.735, 38.005) ccw
  arc A1684 (39.735, 37.8716) -> (39.735, 38.1383) centre (39.735, 38.005) ccw
  arc A1685 (50.735, 38.1383) -> (50.735, 37.8716) centre (50.735, 38.005) ccw
  arc A1686 (39.735, 38.1383) -> (39.735, 37.8716) centre (39.735, 38.005) ccw
  arc A1687 (40.735, 37.8716) -> (40.735, 38.1383) centre (40.735, 38.005) ccw
  arc A1688 (48.735, 37.8716) -> (48.735, 38.1383) centre (48.735, 38.005) ccw
  arc A1689 (49.735, 37.8716) -> (49.735, 38.1383) centre (49.735, 38.005) ccw
  arc A1690 (47.735, 38.1383) -> (47.735, 37.8716) centre (47.735, 38.005) ccw
  arc A1691 (60.735, 38.8716) -> (60.735, 39.1383) centre (60.735, 39.005) ccw
  arc A1692 (60.735, 39.1383) -> (60.735, 38.8716) centre (60.735, 39.005) ccw
  arc A1693 (40.735, 38.1383) -> (40.735, 37.8716) centre (40.735, 38.005) ccw
  arc A1694 (39.735, 38.1383) -> (39.735, 37.8716) centre (39.735, 38.005) ccw
  arc A1695 (41.735, 38.1383) -> (41.735, 37.8716) centre (41.735, 38.005) ccw
  arc A1696 (43.735, 38.1383) -> (43.735, 37.8716) centre (43.735, 38.005) ccw
  arc A1697 (42.735, 37.8716) -> (42.735, 38.1383) centre (42.735, 38.005) ccw
  arc A1698 (45.735, 38.1383) -> (45.735, 37.8716) centre (45.735, 38.005) ccw
  arc A1699 (42.735, 38.1383) -> (42.735, 37.8716) centre (42.735, 38.005) ccw
  arc A1700 (39.735, 37.8716) -> (39.735, 38.1383) centre (39.735, 38.005) ccw
  arc A1701 (42.735, 38.1383) -> (42.735, 37.8716) centre (42.735, 38.005) ccw
  arc A1702 (44.735, 38.1383) -> (44.735, 37.8716) centre (44.735, 38.005) ccw
  arc A1703 (60.735, 39.1383) -> (60.735, 38.8716) centre (60.735, 39.005) ccw
  arc A1704 (41.735, 38.1383) -> (41.735, 37.8716) centre (41.735, 38.005) ccw
  arc A1705 (42.735, 37.8716) -> (42.735, 38.1383) centre (42.735, 38.005) ccw
  arc A1706 (45.735, 37.8716) -> (45.735, 38.1383) centre (45.735, 38.005) ccw
  arc A1707 (40.735, 38.1383) -> (40.735, 37.8716) centre (40.735, 38.005) ccw
  arc A1708 (43.735, 37.8716) -> (43.735, 38.1383) centre (43.735, 38.005) ccw
  arc A1709 (43.735, 38.1383) -> (43.735, 37.8716) centre (43.735, 38.005) ccw
  arc A1710 (42.735, 37.8716) -> (42.735, 38.1383) centre (42.735, 38.005) ccw
  arc A1711 (41.735, 37.8716) -> (41.735, 38.1383) centre (41.735, 38.005) ccw
  arc A1712 (45.735, 37.8716) -> (45.735, 38.1383) centre (45.735, 38.005) ccw
  arc A1713 (47.735, 38.1383) -> (47.735, 37.8716) centre (47.735, 38.005) ccw
  arc A1714 (47.735, 37.8716) -> (47.735, 38.1383) centre (47.735, 38.005) ccw
  arc A1715 (43.735, 37.8716) -> (43.735, 38.1383) centre (43.735, 38.005) ccw
  arc A1716 (47.735, 37.8716) -> (47.735, 38.1383) centre (47.735, 38.005) ccw
  arc A1717 (42.735, 38.1383) -> (42.735, 37.8716) centre (42.735, 38.005) ccw
  arc A1718 (46.735, 37.8716) -> (46.735, 38.1383) centre (46.735, 38.005) ccw
  arc A1719 (57.735, 38.1383) -> (57.735, 37.8716) centre (57.735, 38.005) ccw
  arc A1720 (45.735, 38.1383) -> (45.735, 37.8716) centre (45.735, 38.005) ccw
  arc A1721 (51.735, 37.8716) -> (51.735, 38.1383) centre (51.735, 38.005) ccw
  arc A1722 (52.735, 37.8716) -> (52.735, 38.1383) centre (52.735, 38.005) ccw
  arc A1723 (55.735, 37.8716) -> (55.735, 38.1383) centre (55.735, 38.005) ccw
  arc A1724 (50.735, 37.8716) -> (50.735, 38.1383) centre (50.735, 38.005) ccw
  arc A1725 (47.735, 38.1383) -> (47.735, 37.8716) centre (47.735, 38.005) ccw
  arc A1726 (55.735, 38.1383) -> (55.735, 37.8716) centre (55.735, 38.005) ccw
  arc A1727 (54.735, 37.8716) -> (54.735, 38.1383) centre (54.735, 38.005) ccw
  arc A1728 (54.735, 37.8716) -> (54.735, 38.1383) centre (54.735, 38.005) ccw
  arc A1729 (52.735, 38.1383) -> (52.735, 37.8716) centre (52.735, 38.005) ccw
  arc A1730 (59.735, 37.8716) -> (59.735, 38.1383) centre (59.735, 38.005) ccw
  arc A1731 (60.735, 37.8716) -> (60.735, 38.1383) centre (60.735, 38.005) ccw
  arc A1732 (59.735, 38.1383) -> (59.735, 37.8716) centre (59.735, 38.005) ccw
  arc A1733 (54.735, 38.1383) -> (54.735, 37.8716) centre (54.735, 38.005) ccw
  arc A1734 (59.735, 37.8716) -> (59.735, 38.1383) centre (59.735, 38.005) ccw
  arc A1735 (46.735, 37.8716) -> (46.735, 38.1383) centre (46.735, 38.005) ccw
  arc A1736 (55.735, 38.1383) -> (55.735, 37.8716) centre (55.735, 38.005) ccw
  arc A1737 (57.735, 38.1383) -> (57.735, 37.8716) centre (57.735, 38.005) ccw
  arc A1738 (46.735, 38.1383) -> (46.735, 37.8716) centre (46.735, 38.005) ccw
  arc A1739 (51.735, 37.8716) -> (51.735, 38.1383) centre (51.735, 38.005) ccw
  arc A1740 (44.735, 38.1383) -> (44.735, 37.8716) centre (44.735, 38.005) ccw
  arc A1741 (56.735, 38.1383) -> (56.735, 37.8716) centre (56.735, 38.005) ccw
  arc A1742 (50.735, 38.1383) -> (50.735, 37.8716) centre (50.735, 38.005) ccw
  arc A1743 (52.735, 38.1383) -> (52.735, 37.8716) centre (52.735, 38.005) ccw
  arc A1744 (51.735, 38.1383) -> (51.735, 37.8716) centre (51.735, 38.005) ccw
  arc A1745 (51.735, 38.1383) -> (51.735, 37.8716) centre (51.735, 38.005) ccw
  arc A1746 (60.735, 37.8716) -> (60.735, 38.1383) centre (60.735, 38.005) ccw
  arc A1747 (54.735, 38.1383) -> (54.735, 37.8716) centre (54.735, 38.005) ccw
  arc A1748 (56.735, 38.1383) -> (56.735, 37.8716) centre (56.735, 38.005) ccw
  arc A1749 (51.735, 37.8716) -> (51.735, 38.1383) centre (51.735, 38.005) ccw
  arc A1750 (52.735, 38.1383) -> (52.735, 37.8716) centre (52.735, 38.005) ccw
  arc A1751 (54.735, 38.1383) -> (54.735, 37.8716) centre (54.735, 38.005) ccw
  arc A1752 (51.735, 38.1383) -> (51.735, 37.8716) centre (51.735, 38.005) ccw
  arc A1753 (53.735, 38.1383) -> (53.735, 37.8716) centre (53.735, 38.005) ccw
  arc A1754 (40.735, 37.1384) -> (40.735, 36.8717) centre (40.735, 37.005) ccw
  arc A1755 (58.735, 37.8716) -> (58.735, 38.1383) centre (58.735, 38.005) ccw
  arc A1756 (56.735, 37.8716) -> (56.735, 38.1383) centre (56.735, 38.005) ccw
  arc A1757 (53.735, 37.8716) -> (53.735, 38.1383) centre (53.735, 38.005) ccw
  arc A1758 (52.735, 37.8716) -> (52.735, 38.1383) centre (52.735, 38.005) ccw
  arc A1759 (52.735, 37.8716) -> (52.735, 38.1383) centre (52.735, 38.005) ccw
  arc A1760 (39.735, 37.1384) -> (39.735, 36.8717) centre (39.735, 37.005) ccw
  arc A1761 (59.735, 38.1383) -> (59.735, 37.8716) centre (59.735, 38.005) ccw
  arc A1762 (44.735, 38.1383) -> (44.735, 37.8716) centre (44.735, 38.005) ccw
  arc A1763 (54.735, 37.8716) -> (54.735, 38.1383) centre (54.735, 38.005) ccw
  arc A1764 (53.735, 37.8716) -> (53.735, 38.1383) centre (53.735, 38.005) ccw
  arc A1765 (50.735, 38.1383) -> (50.735, 37.8716) centre (50.735, 38.005) ccw
  arc A1766 (55.735, 37.8716) -> (55.735, 38.1383) centre (55.735, 38.005) ccw
  arc A1767 (56.735, 38.1383) -> (56.735, 37.8716) centre (56.735, 38.005) ccw
  arc A1768 (53.735, 38.1383) -> (53.735, 37.8716) centre (53.735, 38.005) ccw
  arc A1769 (46.735, 37.8716) -> (46.735, 38.1383) centre (46.735, 38.005) ccw
  arc A1770 (53.735, 37.8716) -> (53.735, 38.1383) centre (53.735, 38.005) ccw
  arc A1771 (55.735, 37.8716) -> (55.735, 38.1383) centre (55.735, 38.005) ccw
  arc A1772 (56.735, 37.8716) -> (56.735, 38.1383) centre (56.735, 38.005) ccw
  arc A1773 (48.735, 37.8716) -> (48.735, 38.1383) centre (48.735, 38.005) ccw
  arc A1774 (58.735, 37.8716) -> (58.735, 38.1383) centre (58.735, 38.005) ccw
  arc A1775 (55.735, 38.1383) -> (55.735, 37.8716) centre (55.735, 38.005) ccw
  arc A1776 (56.735, 37.8716) -> (56.735, 38.1383) centre (56.735, 38.005) ccw
  arc A1777 (39.735, 36.8717) -> (39.735, 37.1384) centre (39.735, 37.005) ccw
  arc A1778 (50.735, 37.8716) -> (50.735, 38.1383) centre (50.735, 38.005) ccw
  arc A1779 (44.735, 37.8716) -> (44.735, 38.1383) centre (44.735, 38.005) ccw
  arc A1780 (40.735, 36.8717) -> (40.735, 37.1384) centre (40.735, 37.005) ccw
  arc A1781 (53.735, 38.1383) -> (53.735, 37.8716) centre (53.735, 38.005) ccw
  arc A1782 (58.735, 38.1383) -> (58.735, 37.8716) centre (58.735, 38.005) ccw
  arc A1783 (42.735, 36.8717) -> (42.735, 37.1384) centre (42.735, 37.005) ccw
  arc A1784 (60.735, 38.1383) -> (60.735, 37.8716) centre (60.735, 38.005) ccw
  arc A1785 (43.735, 36.8717) -> (43.735, 37.1384) centre (43.735, 37.005) ccw
  arc A1786 (45.735, 37.1384) -> (45.735, 36.8717) centre (45.735, 37.005) ccw
  arc A1787 (45.735, 37.1384) -> (45.735, 36.8717) centre (45.735, 37.005) ccw
  arc A1788 (44.735, 36.8717) -> (44.735, 37.1384) centre (44.735, 37.005) ccw
  arc A1789 (57.735, 38.1383) -> (57.735, 37.8716) centre (57.735, 38.005) ccw
  arc A1790 (58.735, 38.1383) -> (58.735, 37.8716) centre (58.735, 38.005) ccw
  arc A1791 (42.735, 37.1384) -> (42.735, 36.8717) centre (42.735, 37.005) ccw
  arc A1792 (43.735, 37.1384) -> (43.735, 36.8717) centre (43.735, 37.005) ccw
  arc A1793 (47.735, 36.8717) -> (47.735, 37.1384) centre (47.735, 37.005) ccw
  arc A1794 (43.735, 36.8717) -> (43.735, 37.1384) centre (43.735, 37.005) ccw
  arc A1795 (39.735, 37.1384) -> (39.735, 36.8717) centre (39.735, 37.005) ccw
  arc A1796 (40.735, 37.1384) -> (40.735, 36.8717) centre (40.735, 37.005) ccw
  arc A1797 (41.735, 37.1384) -> (41.735, 36.8717) centre (41.735, 37.005) ccw
  arc A1798 (43.735, 37.1384) -> (43.735, 36.8717) centre (43.735, 37.005) ccw
  arc A1799 (41.735, 36.8717) -> (41.735, 37.1384) centre (41.735, 37.005) ccw
  arc A1800 (60.735, 38.1383) -> (60.735, 37.8716) centre (60.735, 38.005) ccw
  arc A1801 (46.735, 37.1384) -> (46.735, 36.8717) centre (46.735, 37.005) ccw
  arc A1802 (57.735, 37.8716) -> (57.735, 38.1383) centre (57.735, 38.005) ccw
  arc A1803 (42.735, 36.8717) -> (42.735, 37.1384) centre (42.735, 37.005) ccw
  arc A1804 (41.735, 36.8717) -> (41.735, 37.1384) centre (41.735, 37.005) ccw
  arc A1805 (44.735, 37.1384) -> (44.735, 36.8717) centre (44.735, 37.005) ccw
  arc A1806 (42.735, 37.1384) -> (42.735, 36.8717) centre (42.735, 37.005) ccw
  arc A1807 (45.735, 37.1384) -> (45.735, 36.8717) centre (45.735, 37.005) ccw
  arc A1808 (44.735, 37.1384) -> (44.735, 36.8717) centre (44.735, 37.005) ccw
  arc A1809 (47.735, 36.8717) -> (47.735, 37.1384) centre (47.735, 37.005) ccw
  arc A1810 (49.735, 37.1384) -> (49.735, 36.8717) centre (49.735, 37.005) ccw
  arc A1811 (59.735, 37.8716) -> (59.735, 38.1383) centre (59.735, 38.005) ccw
  arc A1812 (60.735, 37.8716) -> (60.735, 38.1383) centre (60.735, 38.005) ccw
  arc A1813 (57.735, 37.8716) -> (57.735, 38.1383) centre (57.735, 38.005) ccw
  arc A1814 (60.735, 38.1383) -> (60.735, 37.8716) centre (60.735, 38.005) ccw
  arc A1815 (46.735, 37.1384) -> (46.735, 36.8717) centre (46.735, 37.005) ccw
  arc A1816 (57.735, 37.8716) -> (57.735, 38.1383) centre (57.735, 38.005) ccw
  arc A1817 (43.735, 36.8717) -> (43.735, 37.1384) centre (43.735, 37.005) ccw
  arc A1818 (42.735, 37.1384) -> (42.735, 36.8717) centre (42.735, 37.005) ccw
  arc A1819 (47.735, 37.1384) -> (47.735, 36.8717) centre (47.735, 37.005) ccw
  arc A1820 (40.735, 36.8717) -> (40.735, 37.1384) centre (40.735, 37.005) ccw
  arc A1821 (39.735, 36.8717) -> (39.735, 37.1384) centre (39.735, 37.005) ccw
  arc A1822 (41.735, 36.8717) -> (41.735, 37.1384) centre (41.735, 37.005) ccw
  arc A1823 (58.735, 37.8716) -> (58.735, 38.1383) centre (58.735, 38.005) ccw
  arc A1824 (44.735, 36.8717) -> (44.735, 37.1384) centre (44.735, 37.005) ccw
  arc A1825 (45.735, 36.8717) -> (45.735, 37.1384) centre (45.735, 37.005) ccw
  arc A1826 (41.735, 37.1384) -> (41.735, 36.8717) centre (41.735, 37.005) ccw
  arc A1827 (45.735, 36.8717) -> (45.735, 37.1384) centre (45.735, 37.005) ccw
  arc A1828 (42.735, 36.8717) -> (42.735, 37.1384) centre (42.735, 37.005) ccw
  arc A1829 (44.735, 37.1384) -> (44.735, 36.8717) centre (44.735, 37.005) ccw
  arc A1830 (47.735, 37.1384) -> (47.735, 36.8717) centre (47.735, 37.005) ccw
  arc A1831 (40.735, 36.8717) -> (40.735, 37.1384) centre (40.735, 37.005) ccw
  arc A1832 (39.735, 37.1384) -> (39.735, 36.8717) centre (39.735, 37.005) ccw
  arc A1833 (46.735, 36.8717) -> (46.735, 37.1384) centre (46.735, 37.005) ccw
  arc A1834 (58.735, 38.1383) -> (58.735, 37.8716) centre (58.735, 38.005) ccw
  arc A1835 (59.735, 38.1383) -> (59.735, 37.8716) centre (59.735, 38.005) ccw
  arc A1836 (46.735, 36.8717) -> (46.735, 37.1384) centre (46.735, 37.005) ccw
  arc A1837 (43.735, 37.1384) -> (43.735, 36.8717) centre (43.735, 37.005) ccw
  arc A1838 (41.735, 37.1384) -> (41.735, 36.8717) centre (41.735, 37.005) ccw
  arc A1839 (40.735, 37.1384) -> (40.735, 36.8717) centre (40.735, 37.005) ccw
  arc A1840 (45.735, 36.8717) -> (45.735, 37.1384) centre (45.735, 37.005) ccw
  arc A1841 (44.735, 36.8717) -> (44.735, 37.1384) centre (44.735, 37.005) ccw
  arc A1842 (47.735, 36.8717) -> (47.735, 37.1384) centre (47.735, 37.005) ccw
  arc A1843 (46.735, 37.1384) -> (46.735, 36.8717) centre (46.735, 37.005) ccw
  arc A1844 (47.735, 37.1384) -> (47.735, 36.8717) centre (47.735, 37.005) ccw
  arc A1845 (39.735, 36.8717) -> (39.735, 37.1384) centre (39.735, 37.005) ccw
  arc A1846 (46.735, 36.8717) -> (46.735, 37.1384) centre (46.735, 37.005) ccw
  line L3068 (47.895, 52.0775) -> (47.895, 54.3505)
  line L3069 (48.395, 46.3495) -> (48.395, 48.6225)
  line L3070 (47.395, 52.0775) -> (47.395, 54.3505)
  line L3071 (48.395, 52.0775) -> (48.395, 54.3505)
  line L3072 (46.395, 52.0775) -> (46.395, 54.3505)
  line L3073 (46.895, 52.0775) -> (46.895, 54.3505)
  arc A1847 (52.735, 37.1384) -> (52.735, 36.8717) centre (52.735, 37.005) ccw
  arc A1848 (48.735, 37.1384) -> (48.735, 36.8717) centre (48.735, 37.005) ccw
  arc A1849 (48.735, 36.8717) -> (48.735, 37.1384) centre (48.735, 37.005) ccw
  arc A1850 (51.735, 36.8717) -> (51.735, 37.1384) centre (51.735, 37.005) ccw
  line L3074 (48.395, 46.3495) -> (48.395, 48.6225)
  line L3075 (48.395, 46.3495) -> (48.395, 48.6225)
  arc A1851 (49.735, 37.1384) -> (49.735, 36.8717) centre (49.735, 37.005) ccw
  line L3076 (61.3283, 54.598) -> (60.4393, 54.598)
  line L3077 (46.395, 52.0775) -> (46.395, 54.3505)
  line L3078 (46.395, 52.0775) -> (46.395, 54.3505)
  arc A1852 (50.735, 36.8717) -> (50.735, 37.1384) centre (50.735, 37.005) ccw
  arc A1853 (49.735, 36.8717) -> (49.735, 37.1384) centre (49.735, 37.005) ccw
  line L3079 (47.895, 46.3495) -> (47.895, 48.6225)
  arc A1854 (52.735, 37.1384) -> (52.735, 36.8717) centre (52.735, 37.005) ccw
  arc A1855 (48.735, 37.1384) -> (48.735, 36.8717) centre (48.735, 37.005) ccw
  line L3080 (47.395, 46.3495) -> (47.395, 48.6225)